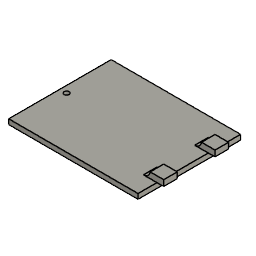
AG07 (Autodesk Fusion 360 design; units mm, degrees)
part number: 2025-10-09-14-04-41-434
Autodesk Fusion 360 part; units mm, degrees
sketch "Boceto1" plane through (0, 0, 0) normal (0, 0, 1) x (1, 0, 0)
  line L0 (-10.8153, 0) -> (-87.4153, 0)
  line L1 (-87.4153, 0) -> (-87.4153, 60.7)
  line L2 (-87.4153, 60.7) -> (-10.8153, 60.7)
  line L3 (-10.8153, 60.7) -> (-10.8153, 0)
  dimension "d1" = 76.6
  dimension "d2" = 60.7
  constraint horizontal L0
  constraint vertical L1
  constraint horizontal L2
  constraint vertical L3
  measures "d1" distance of L1.end L2.end
  measures "d2" distance of L0.end L1.end
extrude "Extruir1" add sketch "Boceto1" along normal blind 3
sketch "Boceto4" plane through (0, 0, 3) normal (0, 0, 1) x (-1, 0, 0)
  line L0 (10.8153, -60.7) -> (87.4153, -60.7)
  line L1 (87.4153, -60.7) -> (87.4153, 0)
  line L2 (87.4153, 0) -> (10.8153, 0)
  line L3 (10.8153, 0) -> (10.8153, -60.7)
  line L4 (10.8153, 0) -> (10.8153, -60.7) construction
  line L5 (10.8153, -30.35) -> (87.4153, -30.35) construction
  line L6 (10.8153, -30.35) -> (10.8153, -60.7) construction
  line L7 (10.8153, -45.525) -> (14.8153, -45.525) construction
  line L8 (14.8153, -45.525) -> (10.8153, -45.525) construction
  line L9 (10.8153, -45.525) -> (10.8153, -41.525) construction
  line L10 (10.8153, -41.525) -> (14.8153, -41.525)
  line L11 (14.8153, -41.525) -> (14.8153, -45.525)
  line L12 (14.8153, -45.525) -> (10.8153, -45.525) construction
  line L13 (10.8153, -45.525) -> (10.8153, -49.525) construction
  line L14 (10.8153, -49.525) -> (14.8153, -49.525)
  line L15 (14.8153, -49.525) -> (14.8153, -45.525)
  line L16 (10.8153, -11.175) -> (14.8153, -11.175)
  line L17 (14.8153, -11.175) -> (14.8153, -15.175)
  line L18 (14.8153, -19.175) -> (14.8153, -15.175)
  line L19 (10.8153, -19.175) -> (14.8153, -19.175)
  dimension "d26" = 4
  dimension "d27" = 4
  dimension "d28" = 4
  constraint coincident L2.end L3.start
  constraint coincident L0.start L3.end
  constraint midpoint L3 L5.start
  constraint midpoint L1 L5.end
  constraint midpoint L6 L7.start
  constraint perpendicular L3 L7
  constraint horizontal L8
  constraint vertical L9
  constraint horizontal L10
  constraint vertical L11
  constraint horizontal L12
  constraint vertical L13
  constraint horizontal L14
  constraint vertical L15
  constraint symmetric L5 L7.end L17.end
  constraint symmetric L5 L9.end L19.start
  constraint symmetric L5 L10.end L18.start
  constraint symmetric L5 L13.end L16.start
  constraint symmetric L5 L14.end L16.end
  measures "d26" distance of L7.start L7.end
  measures "d27" distance of L7.end L10.end
  measures "d28" distance of L7.end L14.end
extrude "Extruir6" add sketch "Boceto4" along normal blind 3.5 contours L3 L10 L11 L14 L15 | L3 L16 L17 L18 L19
sketch "Boceto5" plane through (-10.8153, 0, 0) normal (1, 0, 0) x (0, 1, 0)
  line L0 (0, 0) -> (60.7, 0)
  line L1 (60.7, 0) -> (60.7, 3)
  line L2 (60.7, 3) -> (49.525, 3)
  line L3 (49.525, 3) -> (49.525, 6.5)
  line L4 (49.525, 6.5) -> (41.525, 6.5)
  line L5 (41.525, 6.5) -> (41.525, 3)
  line L6 (41.525, 3) -> (19.175, 3)
  line L7 (19.175, 3) -> (19.175, 6.5)
  line L8 (19.175, 6.5) -> (11.175, 6.5)
  line L9 (11.175, 6.5) -> (11.175, 3)
  line L10 (11.175, 3) -> (0, 3)
  line L11 (0, 3) -> (0, 0)
  line L12 (11.175, 3) -> (19.175, 3)
  line L13 (41.525, 3) -> (49.525, 3)
  constraint coincident L9.end L10.start
  constraint coincident L6.end L7.start
  constraint coincident L5.end L6.start
  constraint coincident L2.end L3.start
extrude "Extruir7" add sketch "Boceto5" along normal blind 4 contours L7 L8 L9 L12 | L3 L4 L5 L13
fillet "Empalme5" radius 4 1 edges at (-14.8153, 45.525, 3)
fillet "Empalme6" radius 4 1 edges at (-14.8153, 15.175, 3)
sketch "Boceto6" plane through (0, 0, 0) normal (0, 0, -1) x (1, 0, 0)
  line L0 (-87.4153, -60.7) -> (-10.8153, -60.7)
  line L1 (-10.8153, -60.7) -> (-10.8153, 0)
  line L2 (-10.8153, 0) -> (-87.4153, 0)
  line L3 (-87.4153, 0) -> (-87.4153, -60.7)
  line L4 (-87.4153, 0) -> (-87.4153, -60.7) construction
  line L5 (-87.4153, -30.35) -> (-83.4153, -30.35) construction
  circle A0 centre (-83.4153, -30.35) radius 1.5
  dimension "d37" = 4
  dimension "d38" = 3
  constraint coincident L2.end L3.start
  constraint coincident L0.start L3.end
  constraint midpoint L3 L5.start
  constraint perpendicular L4 L5
  constraint coincident L5.end A0.centre
  measures "d37" distance of L5.start L5.end
  measures "d38" diameter of A0
extrude "Extruir8" cut sketch "Boceto6" against normal blind 4 contours A0
sketch "Boceto7" plane through (0, 0, 0) normal (0, 0, -1) x (1, 0, 0)
  circle A0 centre (-83.4153, -30.35) radius 1.5
  line L0 (-87.4153, -60.7) -> (-10.8153, -60.7)
  line L1 (-10.8153, -60.7) -> (-10.8153, 0)
  line L2 (-10.8153, 0) -> (-87.4153, 0)
  line L3 (-87.4153, 0) -> (-87.4153, -60.7)
  circle A1 centre (-83.4153, -30.35) radius 2.25
  dimension "d41" = 4.5
  constraint concentric A0 A1
  measures "d41" diameter of A1
extrude "Extruir9" cut sketch "Boceto7" against normal blind 1 contours A1
